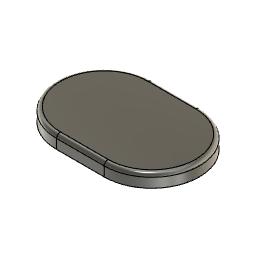
led_diffuser (Autodesk Fusion 360 design; units mm, degrees)
Autodesk Fusion 360 part; units mm, degrees
sketch "Sketch1" plane through (0, 0, 0) normal (0, 0, 1) x (1, 0, 0)
  line L0 (-30, 13) -> (-30, 5) construction
  line L1 (-25, 13) -> (-25, 5) construction
  line L2 (-32, 6) -> (-22, 6) construction
  line L3 (-28.75, 6) -> (-26.25, 6)
  line L4 (-26.2078, 8.4993) -> (-28.7496, 8.5)
  arc A0 (-26.25, 6) -> (-26.2915, 8.4993) centre (-26.25, 7.25) ccw
  arc A1 (-28.7496, 8.5) -> (-28.75, 6) centre (-28.75, 7.25) ccw
  line L5 (-28.7496, 9.75) -> (-26.25, 9.75)
  line L6 (-26.25, 4.75) -> (-28.75, 4.75)
  arc A2 (-26.25, 4.75) -> (-26.25, 9.75) centre (-26.25, 7.25) ccw
  arc A3 (-28.7496, 9.75) -> (-28.75, 4.75) centre (-28.75, 7.25) ccw
  dimension "d1" = 5
  dimension "d2" = 1.25
  dimension "d3" = 1.25
  dimension "d4" = 5
  constraint vertical L0
  constraint vertical L1
  constraint perpendicular L1 L2
  constraint tangent L0 A1
  constraint tangent L2 A1
  constraint tangent L1 A0
  constraint tangent L2 A0
  constraint tangent L3 A0
  constraint coincident L4.start A0
  constraint tangent L4 A1
  constraint coincident L4 A0.end
  constraint concentric A1 A3
  constraint tangent L6 A3
  constraint parallel L3 L6
  measures "d1" distance of L0 L1
  measures "d2" radius of A1
  measures "d3" radius of A0
  measures "d4" diameter of A3
extrude "Extrude1" add sketch "Sketch1" along normal blind 0.2
sketch "Sketch2" plane through (0, 0, 0.2) normal (0, 0, 1) x (-1, 0, 0)
  arc A0 (28.7496, -8.5) -> (28.75, -6) centre (28.75, -7.25) ccw
  line L0 (28.7496, -8.5) -> (26.2915, -8.4993)
  arc A1 (26.25, -6) -> (26.2915, -8.4993) centre (26.25, -7.25) ccw
  line L1 (26.25, -6) -> (28.75, -6)
  arc A2 (26.25, -4.75) -> (26.25, -9.75) centre (26.25, -7.25) ccw
  line L2 (26.25, -9.75) -> (28.7496, -9.75)
  arc A3 (28.7496, -9.75) -> (28.75, -4.75) centre (28.75, -7.25) ccw
  line L3 (28.75, -4.75) -> (26.25, -4.75)
extrude "Extrude2" add sketch "Sketch2" along normal blind 0.5 contours A0 L0 A1 L1 | A2 L2 A3 L3
fillet "Fillet1" radius 0.2 4 edges at (-27.5, 4.75, 0.7) (-23.75, 7.25, 0.7) (-27.4998, 9.75, 0.7) (-31.25, 7.2502, 0.7)
